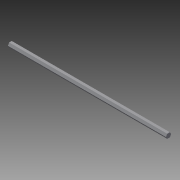
# Autodesk Inventor part: Hexagon Rodpart 2
Saved by Autodesk Inventor 2015 (Build 190159000, 159)
## iProperties
Created: 2015-01-17
Part Number: Hexagon Rodpart 2
Material: Generic
Document SubType Name: Modeling
Designer: whitaus15
Density: 1 g/cm^3
Appearance: Default
Author: whitaus15
Autodesk Inventor part; units mm, degrees
ref_plane "YZ Plane" through (0, 0, 0) normal (1, 0, 0) x (0, 1, 0)
ref_plane "XZ Plane" through (0, 0, 0) normal (0, 1, 0) x (-1, 0, 0)
ref_plane "XY Plane" through (0, 0, 0) normal (0, 0, 1) x (1, 0, 0)
sketch "Sketch1" plane through (0, 0, 0) normal (0, 1, 0) x (-1, 0, 0)
  point P0 (0, 0)
sketch "Sketch2" plane through (0, 0, 0) normal (1, 0, 0) x (0, 1, 0)
  line L0 (1.6165, 4.7349) -> (1.4691, 10.3193)
  line L1 (1.4691, 10.3193) -> (6.2316, 13.2392)
  line L2 (6.2316, 13.2392) -> (11.1415, 10.5747)
  line L3 (11.1415, 10.5747) -> (11.2889, 4.9903)
  line L4 (11.2889, 4.9903) -> (6.5264, 2.0704)
  line L5 (6.5264, 2.0704) -> (1.6165, 4.7349)
  point P0 (0, 0)
  point P1 (6.379, 7.6548)
  dimension "d0" = 9.525
  constraints: 12 end point, 13 other
  measures "d0" horizontal distance of L0.start L2.end
extrude "Extrusion1" add sketch "Sketch2" along normal blind 342.9
body "Solid1"
